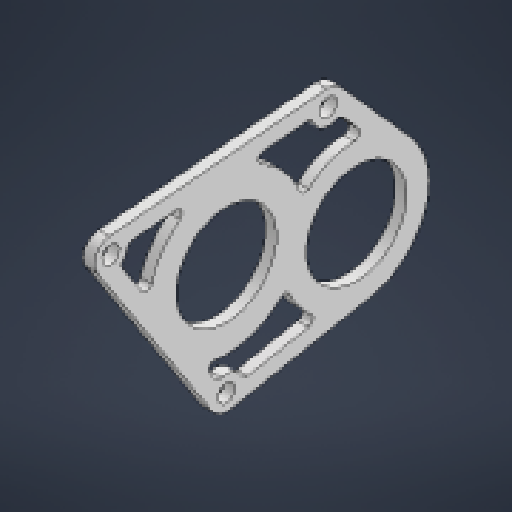
# Autodesk Inventor part: PLATE,BEARING,MOUNT
Saved by Autodesk Inventor 2026.1 (Build 301233020, 233B)
## iProperties
Created: 2026-01-27
Part Number: PLATE,BEARING,MOUNT
Material: Generic
Document SubType Name: Sheet Metal
Designer: Owen L
Density: 1 g/cm^3
Sheet Metal Rule: Default
Appearance: Default
Mass: 9.4797 g
Surface Area: 75.0554 cm^2
Volume: 9.4797 cm^3
Author: Owen L
Autodesk Inventor part; units mm, degrees
ref_plane "YZ Plane" through (0, 0, 0) normal (1, 0, 0) x (0, 1, 0)
ref_plane "XZ Plane" through (0, 0, 0) normal (0, 1, 0) x (-1, 0, 0)
ref_plane "XY Plane" through (0, 0, 0) normal (0, 0, 1) x (1, 0, 0)
sketch "Sketch1" plane through (0, 0, 0) normal (1, 0, 0) x (0, 1, 0)
  line L0 (0, -277.9865) -> (0, 46.3311) construction
  line L1 (36.388, -206.3665) -> (0, 0) construction
  arc A0 (16.1301, -210.3068) -> (50.1142, -221.7774) centre (36.388, -206.3665) ccw
  line L2 (60.8363, -134.6616) -> (44.7346, -169.192) construction
  arc A1 (65.5581, -134.04) -> (58.0495, -130.7996) centre (60.8363, -134.6616) ccw
  arc A2 (72.3924, -201.9346) -> (73.9465, -197.7566) centre (69.2248, -198.3782) ccw
  arc A3 (10.1977, -165.33) -> (8.3097, -170.1013) centre (12.9846, -169.192) ccw
  line L3 (65.5581, -134.04) -> (73.9465, -197.7566)
  line L4 (72.3924, -201.9346) -> (50.1142, -221.7774)
  line L5 (16.1301, -210.3068) -> (8.3097, -170.1013)
  line L6 (69.2248, -198.3782) -> (44.7346, -169.192) construction
  line L7 (58.0495, -130.7996) -> (10.1977, -165.33)
  line L8 (44.7346, -169.192) -> (12.9846, -169.192) construction
  dimension "d8" = 209.55
  dimension "d9" = 175.006
  dimension "d11" = 10
  dimension "d12" = 20.6375
  dimension "d13" = 38.1
  dimension "d14" = 25
  dimension "d19" = 4.7625
  dimension "d37" = 40
  dimension "d39" = 90
  dimension "d40" = 31.75
  dimension "d41" = 38.1
  constraints: 16 end point, 8 point on circle, 8 tangent, 5 coincident, 4 centre point, 2 equal radius, 1 equal length
  measures "d8" distance of L1.end L1.start
  measures "d9" distance of L1.end L2.end
  measures "d11" angle of L0 L1
  measures "d12" radius of A0
  measures "d13" distance of L2.end L2.start
  measures "d14" angle of L0 L2
  measures "d19" radius of A1
  measures "d37" angle of L0 L6
  measures "d39" angle of L0 L8
  measures "d40" distance of L8.start L8.end
  measures "d41" distance of L1.start L2.end
extrude "Plate1" add sketch "Sketch1" along normal blind 3.175
hole "Hole1" at (0, 60.8363, -134.6616) at (0, 12.9846, -169.192) at (0, 69.2248, -198.3782) direction (1, 0, 0) diameter 4.9784 end through all clearance for "Flat Head Machine Screw (82)" size "#10" standard "Ansi Unified Screw Threads"
hole "Hole2" at (0, 36.388, -206.3665) at (0, 44.7346, -169.192) direction (1, 0, 0) diameter 28.575 end through all
sketch "Sketch2" plane through (3.175, 0, 0) normal (1, 0, 0) x (0, 0, -1)
  circle A0 centre (169.192, 44.7346) radius 14.2875 projected
  circle A1 centre (206.3665, 36.388) radius 14.2875 projected
  circle A2 centre (198.3782, 69.2248) radius 2.4892 projected
  circle A3 centre (169.192, 12.9846) radius 2.4892 projected
  circle A4 centre (134.6616, 60.8363) radius 2.4892 projected
  arc A5 (134.04, 65.5581) -> (130.7996, 58.0495) centre (134.6616, 60.8363) ccw projected
  line L0 (165.33, 10.1977) -> (130.7996, 58.0495) projected
  arc A6 (165.33, 10.1977) -> (170.1013, 8.3097) centre (169.192, 12.9846) ccw projected
  line L1 (210.3068, 16.1301) -> (170.1013, 8.3097) projected
  arc A7 (210.3068, 16.1301) -> (221.7774, 50.1142) centre (206.3665, 36.388) ccw projected
  line L2 (201.9346, 72.3924) -> (221.7774, 50.1142) projected
  arc A8 (201.9346, 72.3924) -> (197.7566, 73.9465) centre (198.3782, 69.2248) ccw projected
  line L3 (134.04, 65.5581) -> (197.7566, 73.9465) projected
  line L4 (134.6616, 60.8363) -> (198.3782, 69.2248)
  line L5 (198.3782, 69.2248) -> (218.221, 46.9466)
  arc A9 (209.3975, 20.805) -> (218.221, 46.9466) centre (206.3665, 36.388) ccw
  line L6 (209.3975, 20.805) -> (169.192, 12.9846)
  line L7 (169.192, 12.9846) -> (134.6616, 60.8363)
  circle A10 centre (134.6616, 60.8363) radius 4.7625
  circle A11 centre (198.3782, 69.2248) radius 4.7625
  circle A12 centre (169.192, 12.9846) radius 4.7625
  circle A13 centre (169.192, 44.7346) radius 22.225
  circle A14 centre (206.3665, 36.388) radius 20.6375
  point P0 (0, 0)
  point P1 (196.4534, 18.2872)
  point P2 (186.5015, 30.7943)
  point P3 (161.2634, 23.9719)
  point P4 (166.4051, 16.8466)
  point P5 (173.8668, 13.8939)
  point P6 (190.7995, 49.937)
  point P7 (209.4503, 56.7938)
  point P8 (201.5458, 65.6684)
  point P9 (193.6565, 68.6032)
  point P10 (175.0995, 66.1601)
  point P11 (146.9886, 43.7537)
  point P12 (157.9404, 63.901)
  point P13 (139.3834, 61.458)
  point P14 (137.4485, 56.9744)
  dimension "d42" = 4.7625
  dimension "d44" = 41.275
  dimension "d45" = 44.45
  constraints: 8 end point, 6 centre point, 5 coincident, 3 concentric, 2 point on circle, 4 other
  measures "d42" distance between parallel lines of L0 L7
  measures "d44" diameter of A14
  measures "d45" diameter of A13
extrude "Cut1" cut sketch "Sketch2" against normal blind 3.175 contours A11 L5 A14 A13 L4 | A13 L7 A10 L4 | A14 L6 A12 L7 A13
fillet "Corner Round1" radius 1.5875 14 edges at (1.5875, 43.7537, -146.9886) (1.5875, 63.901, -157.9404) (1.5875, 56.9744, -137.4485) (1.5875, 56.7938, -209.4503) (1.5875, 30.7943, -186.5015) (1.5875, 13.8939, -173.8668) (1.5875, 18.2872, -196.4534) (1.5875, 49.937, -190.7995) (1.5875, 61.458, -139.3834) (1.5875, 68.6032, -193.6565) (1.5875, 65.6684, -201.5458) (1.5875, 66.1601, -175.0995) (1.5875, 16.8466, -166.4051) (1.5875, 23.9719, -161.2634)
equation "\"d25\" = Thickness"
equation "\"d46\" = Thickness"
equation "\"d7\" = Thickness"
equation "\"BendRadius\" = Thickness"
equation "\"BendReliefWidth\" = Thickness"
equation "\"BendReliefDepth\" = 0.5 * Thickness"
equation "\"CornerReliefSize\" = 4 * Thickness"
equation "\"MinimumRemnant\" = 2 * Thickness"
equation "\"TransitionRadius\" = BendRadius"
equation "\"JacobiRadiusSize\" = BendRadius"
equation "\"GapSize\" = Thickness"
equation "\"Thickness\" = 3.175"
body "Solid1"
